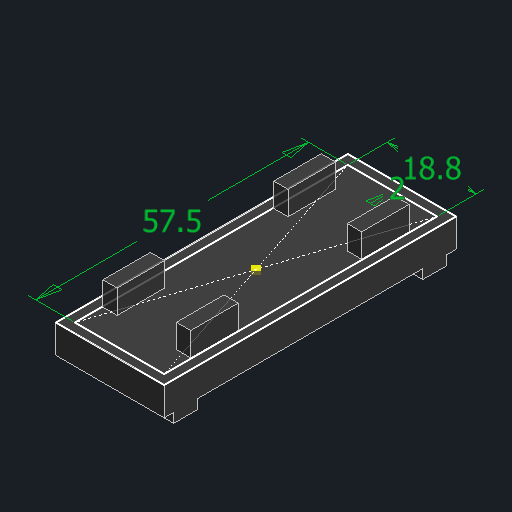
# Autodesk Inventor part: converter2
Saved by Autodesk Inventor 2026.1 (Build 301233020, 233B)
## iProperties
Created: 2025-12-04
Part Number: converter2
Material: 고무, 검은색
Document SubType Name: Modeling
Designer: jaewook
Density: 0.93 g/cm^3
Appearance: 고무 - 검은색
Author: jaewook
Autodesk Inventor part; units mm, degrees
ref_plane "YZ Plane" through (0, 0, 0) normal (1, 0, 0) x (0, 1, 0)
ref_plane "XZ Plane" through (0, 0, 0) normal (0, 1, 0) x (-1, 0, 0)
ref_plane "XY Plane" through (0, 0, 0) normal (0, 0, 1) x (1, 0, 0)
sketch "스케치1" plane through (0, 0, 0) normal (0, 1, 0) x (-1, 0, 0)
  line L0 (-9.4, 28.75) -> (9.4, 28.75)
  line L1 (9.4, 28.75) -> (9.4, -28.75)
  line L2 (9.4, -28.75) -> (-9.4, -28.75)
  line L3 (-9.4, -28.75) -> (-9.4, 28.75)
  line L4 (-9.4, 28.75) -> (9.4, -28.75) construction
  line L5 (9.4, 28.75) -> (-9.4, -28.75) construction
  line L6 (-11.4, -30.75) -> (11.4, -30.75)
  line L7 (11.4, -30.75) -> (11.4, 30.75)
  line L8 (11.4, 30.75) -> (-11.4, 30.75)
  line L9 (-11.4, 30.75) -> (-11.4, -30.75)
  point P0 (0, 0)
  dimension "d0" = 18.8
  dimension "d1" = 57.5
  dimension "d2" = 2
  constraints: 20 end point, 4 parallel, 2 midpoint, 2 perpendicular, 1 horizontal, 3 other
  measures "d0" distance of L1.end L2.end
  measures "d1" distance of L0.end L1.end
  measures "d2" distance between parallel lines of L2 L6
extrude "돌출1" add sketch "스케치1" against normal blind 2 contours L0 L1 L2 L3
extrude "돌출2" add sketch "스케치1" against normal blind 6
sketch "스케치2" plane through (0, -6, 0) normal (0, -1, 0) x (1, 0, 0)
  line L0 (11.4, -30.75) -> (11.4, 30.75) projected
  line L1 (9.4, 28.75) -> (9.4, -28.75) projected
  line L2 (9.4, -28.75) -> (-9.4, -28.75) projected
  line L3 (11.4, -28.75) -> (9.1, -28.75)
  line L4 (9.1, -28.75) -> (9.1, -23.75)
  line L5 (9.1, -23.75) -> (11.4, -23.75)
  line L6 (11.4, -23.75) -> (11.4, -28.75)
  line L7 (0, 0) -> (0, -17.1125) construction
  line L8 (0, 0) -> (-6.0193, 0) construction
  line L9 (-11.4, -28.75) -> (-9.1, -28.75)
  line L10 (-9.1, -28.75) -> (-9.1, -23.75)
  line L11 (-9.1, -23.75) -> (-11.4, -23.75)
  line L12 (11.4, 28.75) -> (9.1, 28.75)
  line L13 (9.1, 28.75) -> (9.1, 23.75)
  line L14 (9.1, 23.75) -> (11.4, 23.75)
  line L15 (-9.1, 28.75) -> (-9.1, 23.75)
  line L16 (-11.4, 28.75) -> (-9.1, 28.75)
  line L17 (-9.1, 23.75) -> (-11.4, 23.75)
  line L18 (-11.4, 30.75) -> (-11.4, -30.75) projected
  line L19 (-11.4, -28.75) -> (-11.4, -23.75)
  line L20 (-11.4, 23.75) -> (-11.4, 28.75)
  line L21 (11.4, 23.75) -> (11.4, 28.75)
  point P0 (-9.1, -28.75)
  dimension "d7" = 0.3
  dimension "d8" = 5
  constraints: 36 end point, 12 symmetric about line, 4 collinear, 2 horizontal, 2 parallel, 2 vertical, 1 perpendicular
  measures "d7" distance between parallel lines of L1 L4
  measures "d8" distance between parallel lines of L5 L3
extrude "돌출3" add sketch "스케치2" along normal blind 2 contours L3 L1 L5 L0 | L18 L16 L15 L17 | L2 L9 L18 L11 L10 | L2 L4 L5 L1 | L14 L1 L12 L0 | L14 L13 L12 L1
sketch "스케치3" plane through (0, 0, 0) normal (0, 1, 0) x (1, 0, 0)
  line L0 (6.25, -23) -> (-6.25, -23)
  line L1 (-6.25, -23) -> (-6.25, 23)
  line L2 (-6.25, 23) -> (6.25, 23)
  line L3 (6.25, 23) -> (6.25, -23)
  line L4 (6.25, -23) -> (-6.25, 23) construction
  line L5 (-6.25, -23) -> (6.25, 23) construction
  line L6 (0, -23) -> (0, 23) construction
  line L7 (9.4, -23.75) -> (9.4, 23.75) construction
  line L8 (9.4, 0) -> (-6.25, 0) construction
  line L9 (-6.25, -23) -> (-9.25, -23)
  line L10 (-9.25, -23) -> (-9.25, -13)
  line L11 (-9.25, -13) -> (-6.25, -13)
  line L12 (-6.25, -13) -> (-6.25, -23)
  line L13 (6.25, -23) -> (9.25, -23)
  line L14 (9.25, -23) -> (9.25, -13)
  line L15 (9.25, -13) -> (6.25, -13)
  line L16 (6.25, -13) -> (6.25, -23)
  line L17 (-6.25, 23) -> (-9.25, 23)
  line L18 (-9.25, 23) -> (-9.25, 13)
  line L19 (-9.25, 13) -> (-6.25, 13)
  line L20 (-6.25, 13) -> (-6.25, 23)
  line L21 (9.25, 13) -> (6.25, 13)
  line L22 (6.25, 13) -> (6.25, 23)
  line L23 (9.25, 23) -> (9.25, 13)
  line L24 (6.25, 23) -> (9.25, 23)
  point P0 (0, 0)
  dimension "d12" = 46
  dimension "d13" = 3
  dimension "d14" = 10
  dimension "d15" = 9.25
  constraints: 48 end point, 9 symmetric about line, 5 midpoint, 4 parallel, 2 horizontal, 2 perpendicular, 2 other
  measures "d12" distance between parallel lines of L2 L0
  measures "d13" distance of L10.end L11.end
  measures "d14" distance of L9.end L10.end
  measures "d15" distance between parallel lines of L6 L10
extrude "돌출4" add sketch "스케치3" along normal blind 5 contours L3 L15 L14 L13 | L9 L10 L11 L1 | L3 L24 L23 L21 | L19 L18 L17 L1
